Side Cover (Autodesk Fusion 360 design; units mm, degrees)
Autodesk Fusion 360 part; units mm, degrees
sketch "Sketch2" plane through (0, 0, 0) normal (0, 0, 1) x (1, 0, 0)
  line L0 (-214.5, -61) -> (-214.5, 61)
  line L1 (-214.5, -61) -> (214.5, 61) construction
  line L2 (-214.5, 61) -> (214.5, 61)
  circle A0 centre (42.5, -3.3) radius 4.1
  line L3 (214.5, -61) -> (-214.5, 61) construction
  line L4 (214.5, 61) -> (214.5, -61)
  line L5 (214.5, -61) -> (-214.5, -61)
  line L6 (-214.5, 0) -> (214.5, 0) construction
  line L7 (-214.5, -3.3) -> (214.5, -3.3) construction
  line L8 (42.5, 61) -> (42.5, -61) construction
  circle A1 centre (42.5, 51) radius 2.1
  line L9 (-214.5, 51) -> (214.5, 51) construction
  circle A2 centre (42.5, -3.3) radius 22.5 construction
  circle A3 centre (42.5, 19.2) radius 2.1
  circle A4 centre (23.0144, 7.95) radius 2.1
  circle A5 centre (23.0144, -14.55) radius 2.1
  circle A6 centre (42.5, -25.8) radius 2.1
  circle A7 centre (61.9856, -14.55) radius 2.1
  circle A8 centre (61.9856, 7.95) radius 2.1
  line L10 (-194.5, 61) -> (-194.5, -61) construction
  line L11 (194.5, 61) -> (194.5, -61) construction
  circle A9 centre (-167.5, 51) radius 2.1
  circle A10 centre (-97.5, 51) radius 2.1
  circle A11 centre (-27.5, 51) radius 2.1
  circle A12 centre (112.5, 51) radius 2.1
  circle A13 centre (182.5, 51) radius 2.1
  circle A14 centre (112.5, -51) radius 2.1
  line L12 (-214.5, -51) -> (214.5, -51) construction
  circle A15 centre (-27.5, -51) radius 2.1
  circle A16 centre (-167.5, -51) radius 2.1
  circle A17 centre (182.5, -51) radius 2.1
  circle A18 centre (-97.5, -51) radius 2.1
  circle A19 centre (42.5, -51) radius 2.1
  circle A20 centre (-204.5, 0) radius 2.1
  circle A21 centre (204.5, 0) radius 2.1
  dimension "d11" = 122
  dimension "d12" = 429
  dimension "d14" = 8.2
  dimension "d18" = 3.3
  dimension "d20" = 172
  dimension "d21" = 4.2
  dimension "d23" = 10
  dimension "d24" = 45
  dimension "d25" = 4.2
  dimension "d27" = 360
  dimension "d30" = 70
  dimension "d31" = 0
  dimension "d32" = 20
  dimension "d33" = 20
  dimension "d34" = 4.2
  dimension "d35" = 10
  dimension "d36" = 4.2
  dimension "d37" = 10
  constraint perpendicular L0 L5
  constraint parallel L2 L5
  constraint parallel L0 L4
  constraint horizontal L5
  constraint coincident origin L3
  constraint coincident origin L1
  constraint midpoint L0 L6.start
  constraint midpoint L4 L6.end
  constraint coincident A0.centre L7
  constraint coincident L2 L8.start
  constraint coincident L5 L8.end
  constraint perpendicular L5 L8
  constraint coincident A0.centre L8
  constraint coincident L8 A1.centre
  constraint coincident L0 L9.start
  constraint coincident L4 L9.end
  constraint perpendicular L4 L9
  constraint coincident A1.centre L9
  constraint concentric A0 A2
  constraint coincident A2 A3.centre
  constraint coincident L8 A3.centre
  constraint coincident L2 L10.start
  constraint coincident L5 L10.end
  constraint perpendicular L5 L10
  constraint coincident L2 L11.start
  constraint coincident L5 L11.end
  constraint perpendicular L5 L11
  constraint symmetric L6 A1 A19
  constraint symmetric L6 L9.start L12.start
  constraint symmetric L6 L9.end L12.end
  constraint symmetric L6 A9 A16
  constraint symmetric L6 A10 A18
  constraint symmetric L6 A11 A15
  constraint symmetric L6 A12 A14
  constraint symmetric L6 A13 A17
  constraint coincident L6 A20.centre
  constraint coincident L6 A21.centre
  measures "d11" distance of L0.start L0.end
  measures "d12" distance of L0.end L1.end
  measures "d14" diameter of A0
  measures "d20" distance of L1.end L8.start
  measures "d21" diameter of A1
  measures "d23" distance of L1.end L9.end
  measures "d24" diameter of A2
  measures "d25" diameter of A3
  measures "d32" distance of L0 L10
  measures "d33" distance of L4 L11
  measures "d34" diameter of A20
  measures "d35" distance of L6.start A20.centre
  measures "d36" diameter of A21
  measures "d37" distance of L6.end A21.centre
extrude "Extrude2" add sketch "Sketch2" along normal blind 3.5
sketch "Sketch3" plane through (0, 0, 3.5) normal (0, 0, 1) x (-1, 0, 0)
  circle A0 centre (-42.5, 3.3) radius 4
  line L0 (-214.5, 61) -> (-214.5, -61)
  line L1 (-214.5, -61) -> (214.5, -61)
  line L2 (214.5, -61) -> (214.5, 61)
  line L3 (214.5, 61) -> (-214.5, 61)
  line L4 (-130, -50) -> (-141.5967, -50) construction
  line L5 (-141.5967, -50) -> (-141.5967, -60) construction
  line L6 (-141.5967, -60) -> (-130, -60) construction
  line L7 (-130, -60) -> (-130, -50) construction
  circle A1 centre (-182.5, 51) radius 2.1
  circle A2 centre (97.5, 51) radius 2.1
  circle A3 centre (-42.5, 51) radius 2.1
  circle A4 centre (204.5, 0) radius 2.1
  circle A5 centre (-204.5, 0) radius 2.1
  circle A6 centre (167.5, 51) radius 2.1
  circle A7 centre (97.5, -51) radius 2.1
  circle A8 centre (27.5, -51) radius 2.1
  circle A9 centre (-112.5, -51) radius 2.1
  circle A10 centre (-182.5, -51) radius 2.1
  circle A11 centre (-112.5, 51) radius 2.1
  circle A12 centre (27.5, 51) radius 2.1
  circle A13 centre (167.5, -51) radius 2.1
  circle A14 centre (-61.9856, -7.95) radius 2.1
  circle A15 centre (-61.9856, 14.55) radius 2.1
  circle A16 centre (-42.5, 25.8) radius 2.1
  circle A17 centre (-23.0144, 14.55) radius 2.1
  circle A18 centre (-23.0144, -7.95) radius 2.1
  circle A19 centre (-42.5, -19.2) radius 2.1
  circle A20 centre (-42.5, -51) radius 2.1
  circle A21 centre (-42.5, 3.3) radius 4.1
  line L8 (-214.5, 61) -> (-214.5, -61)
  line L9 (-214.5, -61) -> (214.5, -61)
  line L10 (214.5, -61) -> (214.5, 61)
  line L11 (214.5, 61) -> (-214.5, 61)
  constraint perpendicular L4 L5
  constraint parallel L4 L6
  constraint parallel L5 L7
